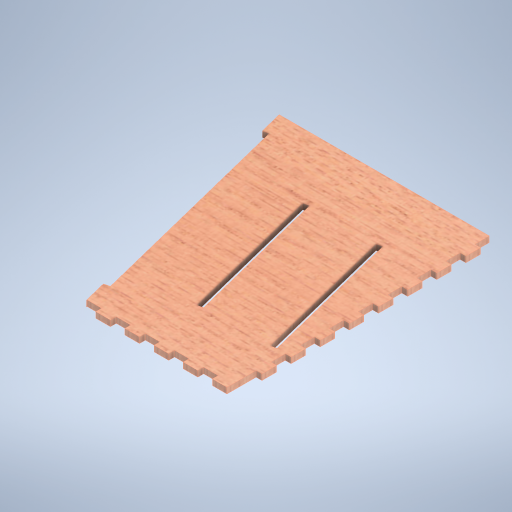
# Autodesk Inventor part: ER_lipo_side_2
Saved by Autodesk Inventor 2023 (Build 270158000, 158)
## iProperties
Created: 2023-03-05
Part Number: ER_lipo_side_2
Material: 木材 (オーク)
Document SubType Name: Modeling
Designer: mkhr7
Density: 0.76 g/cm^3
Appearance: ホワイト オーク材 - ナチュラル 標準の光沢
Author: mkhr7
Autodesk Inventor part; units mm, degrees
ref_plane "YZ Plane" through (0, 0, 0) normal (1, 0, 0) x (0, 1, 0)
ref_plane "XZ Plane" through (0, 0, 0) normal (0, 1, 0) x (-1, 0, 0)
ref_plane "XY Plane" through (0, 0, 0) normal (0, 0, 1) x (1, 0, 0)
sketch "スケッチ1" plane through (0, 0, 0) normal (0, 1, 0) x (-1, 0, 0)
  line L0 (0, 0) -> (100, 0)
  line L1 (100, 0) -> (100, -180)
  line L2 (100, -180) -> (0, -180)
  line L3 (0, -180) -> (0, 0)
  line L4 (0, -170) -> (-4, -170)
  line L5 (-4, -170) -> (-4, -160)
  line L6 (-4, -160) -> (0, -160)
  line L7 (0, -160) -> (0, -170)
  line L8 (-4, -140) -> (0, -140)
  line L9 (-4, -150) -> (-4, -140)
  line L10 (0, -150) -> (-4, -150)
  line L11 (-4, -120) -> (0, -120)
  line L12 (-4, -130) -> (-4, -120)
  line L13 (0, -130) -> (-4, -130)
  line L14 (-4, -100) -> (0, -100)
  line L15 (-4, -110) -> (-4, -100)
  line L16 (0, -110) -> (-4, -110)
  line L17 (-4, -80) -> (0, -80)
  line L18 (-4, -90) -> (-4, -80)
  line L19 (0, -90) -> (-4, -90)
  line L20 (-4, -60) -> (0, -60)
  line L21 (-4, -70) -> (-4, -60)
  line L22 (0, -70) -> (-4, -70)
  line L23 (-4, -40) -> (0, -40)
  line L24 (-4, -50) -> (-4, -40)
  line L25 (0, -50) -> (-4, -50)
  line L26 (-4, -20) -> (0, -20)
  line L27 (-4, -30) -> (-4, -20)
  line L28 (0, -30) -> (-4, -30)
  line L29 (10, 0) -> (20, 0)
  line L30 (20, 0) -> (20, 4)
  line L31 (20, 4) -> (10, 4)
  line L32 (10, 4) -> (10, 0)
  line L33 (30, 4) -> (30, 0)
  line L34 (40, 4) -> (30, 4)
  line L35 (40, 0) -> (40, 4)
  line L36 (50, 4) -> (50, 0)
  line L37 (60, 4) -> (50, 4)
  line L38 (60, 0) -> (60, 4)
  line L39 (70, 4) -> (70, 0)
  line L40 (80, 4) -> (70, 4)
  line L41 (80, 0) -> (80, 4)
  line L42 (45, -180) -> (5, -20)
  line L43 (90.5, -180) -> (50.5, -20)
  line L44 (100, -20) -> (140, -180)
  line L45 (100, -180) -> (140, -180)
  line L46 (100, -3.5076) -> (144.2959, -180.6913)
  line L47 (140, -180) -> (144.1231, -180)
  line L48 (50.5, -20) -> (54.3806, -19.0299)
  line L49 (54.3806, -19.0299) -> (94.6231, -180)
  line L50 (5, -20) -> (1.1194, -20.9701)
  line L51 (1.1194, -20.9701) -> (40.8769, -180)
  line L52 (34.1043, -136.4171) -> (30.2237, -137.3872)
  line L53 (9.8507, -39.4029) -> (5.9701, -40.373)
  line L54 (55.3507, -39.4029) -> (59.2313, -38.4327)
  line L55 (79.6043, -136.4171) -> (83.4848, -135.447)
  line L56 (100, -20) -> (103.8806, -19.0299)
  line L57 (103.8806, -19.0299) -> (140.2609, -164.5512)
  line L58 (140.2609, -164.5512) -> (136.3803, -165.5214)
  line L59 (20, 0) -> (20, -4)
  line L60 (10, -4) -> (10, 0)
  line L61 (30, -4) -> (30, 0)
  line L62 (40, -4) -> (30, -4)
  line L63 (40, 0) -> (40, -4)
  line L64 (50, -4) -> (50, 0)
  line L65 (60, 0) -> (60, -4)
  line L66 (70, -4) -> (70, 0)
  line L67 (80, 0) -> (80, -4)
  line L68 (80, -4) -> (70, -4)
  line L69 (60, -4) -> (50, -4)
  line L70 (20, -4) -> (10, -4)
  line L71 (90, 0) -> (100, 0)
  line L72 (100, 0) -> (100, -4)
  line L73 (100, -4) -> (90, -4)
  line L74 (90, -4) -> (90, 0)
  point P0 (10, 2)
  point P1 (30, 2)
  point P2 (50, 2)
  point P3 (70, 2)
  point P4 (57.291, -38.9178)
  point P5 (0, -20)
  point P6 (0, -40)
  point P7 (0, -60)
  point P8 (0, -80)
  point P9 (0, -100)
  point P10 (0, -120)
  point P11 (0, -140)
  point P12 (0, -160)
  point P13 (50, -2)
  dimension "d0" = 100
  dimension "d1" = 180
  dimension "d2" = 4
  dimension "d3" = 10
  dimension "d4" = 10
  dimension "d7" = 20
  dimension "d12" = 10
  dimension "d13" = 4
  dimension "d14" = 10
  dimension "d17" = 20
  dimension "d22" = 45
  dimension "d23" = 5
  dimension "d24" = 20
  dimension "d26" = 45.5
  dimension "d27" = 45.5
  dimension "d28" = 20
  dimension "d29" = 49.5
  dimension "d30" = 49.5
  dimension "d32" = 4
  dimension "d33" = 4
  dimension "d34" = 4
  dimension "d35" = 20
  dimension "d36" = 100
  dimension "d37" = 20
  dimension "d38" = 100
  dimension "d39" = 150
  dimension "d42" = 10
  dimension "d43" = 4
  dimension "d44" = 10
  constraints: 150 end point, 20 point on line, 12 perpendicular, 10 parallel, 9 symmetric about line, 7 horizontal, 2 collinear, 2 midpoint, 1 vertical, 73 other
  measures "d0" distance of L1.end L2.end
  measures "d1" distance of L0.end L1.end
  measures "d2" distance of L5.end L6.end
  measures "d3" distance of L4.end L5.end
  measures "d4" distance between parallel lines of L2 L4
  measures "d7" distance of L5.end L8.start
  measures "d12" distance of L31.end L30.end
  measures "d13" distance of L30.end L29.end
  measures "d14" distance from line of point (10, 2) L3
  measures "d17" distance of L31.end L33.start
  measures "d22" distance of L42.start L2.end
  measures "d23" distance from line of L3 L42.end
  measures "d24" vertical distance of L0.start L42.end
  measures "d26" distance of L42.start L43.start
  measures "d27" distance of L43.end L42.end
  measures "d28" distance from line of L0 L43.end
  measures "d29" distance of L44.start L43.end
  measures "d30" distance of L44.end L43.start
  measures "d32" distance between parallel lines of L46 L44
  measures "d33" distance of L43.end L48.end
  measures "d34" distance of L42.end L50.end
  measures "d35" distance between parallel lines of L50 L53
  measures "d36" distance between parallel lines of L53 L52
  measures "d37" distance from line of L48 point (57.291, -38.918)
  measures "d38" distance between parallel lines of L55 L54
  measures "d39" distance of L56.end L57.end
  measures "d42" distance of L72.end L73.end
  measures "d43" distance of L71.end L72.end
  measures "d44" distance between parallel lines of L74 L67
extrude "押し出し1" add sketch "スケッチ1" along normal blind 4 contours L0 L60 L70 L59 L61 L62 L63 L64 L69 L65 L66 L68 L67 L74 L73 L1 L2 L49 L48 L43 L42 L50 L51 L3 | L3 L28 L27 L26 | L3 L25 L24 L23 | L3 L22 L21 L20 | L3 L19 L18 L17 | L3 L16 L15 L14 | L46 L56 L1 | L3 L13 L12 L11 | L44 L45 L1 | L46 L47 L44 L58 | L3 L10 L9 L8 | L2 L43 L55 L49 | L3 L4 L5 L6 | L2 L51 L52 L42 | L54 L43 L48 L49 | L53 L51 L50 L42
